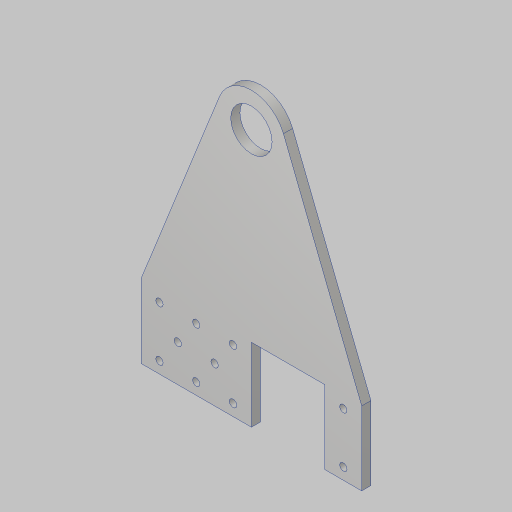
# Autodesk Inventor part: CL3-004
Saved by Autodesk Inventor 2023.5 (Build 275446000, 446)
## iProperties
Created: 2025-01-28
Part Number: CL3-004
Material: Aluminum 6061
Document SubType Name: Modeling
Designer: slick
Density: 2.7 g/cm^3
Appearance: Aluminum - Flat
Mass: 311.171 g
Surface Area: 423.623 cm^2
Volume: 115.249 cm^3
Author: slick
Autodesk Inventor part; units mm, degrees
ref_plane "YZ Plane" through (0, 0, 0) normal (1, 0, 0) x (0, 1, 0)
ref_plane "XZ Plane" through (0, 0, 0) normal (0, 1, 0) x (-1, 0, 0)
ref_plane "XY Plane" through (0, 0, 0) normal (0, 0, 1) x (1, 0, 0)
sketch "Sketch1" plane through (0, 0, 0) normal (0, 0, 1) x (1, 0, 0)
  line L0 (-76.2, 25.4) -> (76.2, 25.4) construction
  line L1 (76.2, 25.4) -> (76.2, -25.4) construction
  line L2 (76.2, -25.4) -> (-76.2, -25.4) construction
  line L3 (-76.2, -25.4) -> (-76.2, 25.4) construction
  line L4 (-76.2, 25.4) -> (76.2, -25.4) construction
  line L5 (76.2, 25.4) -> (-76.2, -25.4) construction
  line L6 (63.5, 17.4625) -> (63.5, -17.4625) construction
  line L7 (9.525, 15.875) -> (41.275, 15.875) construction
  line L8 (41.275, 15.875) -> (41.275, -15.875) construction
  line L9 (41.275, -15.875) -> (9.525, -15.875) construction
  line L10 (9.525, -15.875) -> (9.525, 15.875) construction
  line L11 (9.525, 15.875) -> (41.275, -15.875) construction
  line L12 (41.275, 15.875) -> (9.525, -15.875) construction
  line L13 (76.2, 101.6) -> (187.452, 101.6) construction
  line L14 (187.452, 101.6) -> (187.452, -25.4) construction
  line L15 (187.452, -25.4) -> (76.2, -25.4) construction
  line L16 (76.2, -25.4) -> (76.2, 101.6) construction
  line L17 (76.2, 101.6) -> (187.452, -25.4) construction
  line L18 (187.452, 101.6) -> (76.2, -25.4) construction
  point P0 (0, 0)
  point P1 (63.5, 0)
  point P2 (25.4, 0)
  point P3 (50.8, 0)
  point P4 (0, 0)
  point P5 (9.525, 0)
  point P6 (-12.7, 17.4625)
  point P7 (-12.7, -17.4625)
  point P8 (-25.4, 0)
  point P9 (-38.1, 17.4625)
  point P10 (-38.1, -17.4625)
  point P11 (-50.8, 0)
  point P12 (-63.5, 17.4625)
  point P13 (-63.5, -17.4625)
  point P14 (131.826, 38.1)
  dimension "d0" = 152.4
  dimension "d1" = 50.8
  dimension "d2" = 34.925
  dimension "d3" = 12.7
  dimension "d4" = 31.75
  dimension "d5" = 31.75
  dimension "d6" = 34.925
  dimension "d7" = 25.4
  dimension "d8" = 9.525
  dimension "d9" = 12.7
  dimension "d10" = 12.7
  dimension "d11" = 12.7
  dimension "d12" = 12.7
  dimension "d13" = 12.7
  dimension "d14" = 111.252
  dimension "d15" = 127
  dimension "d16" = 76.2
  constraints: 38 end point, 11 horizontal alignment, 8 midpoint, 6 parallel, 4 vertical alignment, 3 horizontal, 3 perpendicular, 2 coincident, 1 vertical
  measures "d0" distance of L1.end L2.end
  measures "d1" distance of L0.end L1.end
  measures "d2" distance of L6.end L6.start
  measures "d3" distance from line of L1 L6.start
  measures "d4" distance of L8.end L9.end
  measures "d5" distance of L7.end L8.end
  measures "d6" distance between parallel lines of L1 L8
  measures "d7" distance from line of L1 point (50.8, 0)
  measures "d8" distance of point (9.525, 0) point (0, 0)
  measures "d9" horizontal distance of point (0, 0) point (-12.7, 17.463)
  measures "d10" horizontal distance of point (-38.1, 17.463) point (-25.4, 0)
  measures "d11" horizontal distance of point (-38.1, -17.463) point (-50.8, 0)
  measures "d12" horizontal distance of point (-12.7, -17.463) point (-25.4, 0)
  measures "d13" horizontal distance of point (-63.5, 17.463) point (-50.8, 0)
  measures "d14" distance of L14.end L15.end
  measures "d15" distance of L13.end L14.end
  measures "d16" distance between parallel lines of L13 L0
sketch "Sketch2" plane through (0, 0, 0) normal (0, 0, 1) x (1, 0, 0)
  line L0 (63.5, 17.4625) -> (63.5, -17.4625) construction
  line L1 (76.2, 25.4) -> (76.2, -25.4) construction
  line L2 (76.2, -25.4) -> (76.2, 101.6) construction
  line L3 (187.452, -25.4) -> (76.2, -25.4) construction
  line L4 (187.452, 101.6) -> (187.452, -25.4) construction
  line L5 (76.2, 101.6) -> (187.452, -25.4) construction
  line L6 (187.452, 101.6) -> (76.2, -25.4) construction
  line L7 (76.2, 101.6) -> (187.452, 101.6) construction
  line L8 (9.525, 15.875) -> (41.275, 15.875) construction
  line L9 (41.275, 15.875) -> (41.275, -15.875) construction
  line L10 (41.275, -15.875) -> (9.525, -15.875) construction
  line L11 (9.525, -15.875) -> (9.525, 15.875) construction
  line L12 (9.525, 15.875) -> (41.275, -15.875) construction
  line L13 (41.275, 15.875) -> (9.525, -15.875) construction
  line L14 (-76.2, 25.4) -> (76.2, 25.4) construction
  line L15 (76.2, -25.4) -> (-76.2, -25.4) construction
  line L16 (-76.2, 25.4) -> (76.2, -25.4) construction
  line L17 (76.2, 25.4) -> (-76.2, -25.4) construction
  line L18 (-76.2, -25.4) -> (-76.2, 25.4) construction
  line L19 (0, 25.4) -> (0, -25.4)
  line L20 (0, -25.4) -> (-76.2, -25.4)
  line L21 (-76.2, -25.4) -> (-76.2, 25.4)
  line L22 (-76.2, 25.4) -> (-22.1232, 161.2091)
  circle A0 centre (0, 152.4) radius 14.2875
  circle A1 centre (0, 152.4) radius 23.8125 construction
  line L23 (22.1232, 161.2091) -> (76.2, 25.4)
  line L24 (76.2, 25.4) -> (76.2, -25.4)
  line L25 (76.2, -25.4) -> (50.8, -25.4)
  line L26 (50.8, -25.4) -> (50.8, 25.4)
  line L27 (50.8, 25.4) -> (0, 25.4)
  arc A2 (22.1232, 161.2091) -> (-22.1232, 161.2091) centre (0, 152.4) ccw
  point P0 (0, 0)
  point P1 (63.5, 0)
  point P2 (131.826, 38.1)
  point P3 (9.525, 0)
  point P4 (0, 0)
  point P5 (25.4, 0)
  point P6 (-63.5, -17.4625)
  point P7 (-63.5, 17.4625)
  point P8 (-50.8, 0)
  point P9 (-38.1, -17.4625)
  point P10 (-38.1, 17.4625)
  point P11 (-25.4, 0)
  point P12 (-12.7, -17.4625)
  point P13 (-12.7, 17.4625)
  point P14 (0, 0)
  point P15 (50.8, 0)
  point P16 (0, 0)
  dimension "d17" = 28.575
  dimension "d18" = 9.525
  dimension "d19" = 177.8
  dimension "d20" = 9.525
  dimension "d21" = 9.525
  constraints: 18 end point, 4 point on circle, 3 centre point, 3 coincident, 3 midpoint, 2 collinear, 2 point on line, 2 tangent, 1 perpendicular, 1 vertical alignment
  measures "d17" diameter of A0
  measures "d18" radial gap between concentric circles of A0 A1
  measures "d19" distance of L19.end A0.centre
  measures "d20" distance between parallel lines of L11 L19
  measures "d21" distance between parallel lines of L26 L9
extrude "Extrusion1" add sketch "Sketch2" along normal blind 6.35
hole "Hole1" at (76.2, 101.6, 0) at (131.826, 38.1, 0) at (187.452, -25.4, 0) at (9.525, 0, 0) at (9.525, 15.875, 0) at (41.275, -15.875, 0) at (41.275, 15.875, 0) at (9.525, -15.875, 0) at (25.4, 0, 0) at (-63.5, -17.4625, 0) at (-63.5, 17.4625, 0) at (-50.8, 0, 0) at (-38.1, -17.4625, 0) at (-38.1, 17.4625, 0) at (-25.4, 0, 0) at (-12.7, -17.4625, 0) at (-12.7, 17.4625, 0) at (63.5, 17.4625, 0) at (63.5, -17.4625, 0) direction (0, 0, 1) diameter 5.1054 end through all clearance for "Flat Head Machine Screw (82)" size "#10" standard "Ansi Unified Screw Threads"
body "Solid1"
